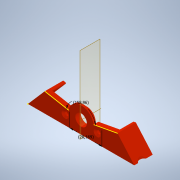
# Autodesk Inventor part: pizza_2
Saved by Autodesk Inventor 2022 (Build 260153000, 153)
## iProperties
Created: 2022-07-28
Part Number: pizza_2
Material: Типовые
Document SubType Name: Modeling
Designer: akapu
Density: 1 g/cm^3
Appearance: По умолчанию
Author: akapu
Autodesk Inventor part; units mm, degrees
ref_plane "YZ Plane" through (0, 0, 0) normal (1, 0, 0) x (0, 1, 0)
ref_plane "XZ Plane" through (0, 0, 0) normal (0, 1, 0) x (-1, 0, 0)
sketch "Эскиз1" plane through (0, 0, 0) normal (0, 0, 1) x (1, 0, 0)
  line L0 (0, 0) -> (35.556, 0)
  line L1 (35.556, 0) -> (57.84, 0)
  line L2 (57.84, 0) -> (93.396, 0)
  line L3 (0, 0) -> (67.4393, 0) construction
  line L4 (35.556, 0) -> (57.84, 0)
  line L5 (46.698, 0) -> (46.698, 11.142)
  line L6 (35.556, 0) -> (35.556, 11.142)
  line L7 (57.84, 0) -> (57.84, 11.142)
  circle A0 centre (46.698, 11.142) radius 11.142
  circle A1 centre (46.698, 11.142) radius 28
  line L8 (0, 0) -> (25.5349, 29.4757)
  line L9 (93.396, 0) -> (67.8611, 29.4757)
  line L10 (46.698, 11.142) -> (31.398, 11.142)
  line L11 (46.698, 11.142) -> (61.998, 11.142)
  circle A2 centre (31.398, 11.142) radius 1.6
  circle A3 centre (61.998, 11.142) radius 1.6
  line L12 (46.698, 11.142) -> (66.497, 30.941)
  line L13 (46.698, 11.142) -> (74.698, 11.142) construction
  line L14 (46.698, 11.142) -> (26.899, 30.941)
  line L15 (46.698, 11.142) -> (74.698, 11.142) construction
  line L16 (46.698, 11.142) -> (19.1687, 16.2546)
  line L17 (46.698, 11.142) -> (74.2273, 16.2546)
  line L18 (19.1687, 16.2546) -> (14.7865, 17.0684)
  line L19 (74.2273, 16.2546) -> (78.6095, 17.0684)
  point P0 (54.5766, 19.0206)
  point P1 (38.8194, 19.0206)
  point P2 (35.7433, 13.1764)
  point P3 (57.6527, 13.1764)
  dimension "d0" = 35.556
  dimension "d1" = 22.284
  dimension "d2" = 35.556
  dimension "d5" = 11.142
  dimension "d6" = 56
  dimension "d7" = 15.3
  dimension "d8" = 15.3
  dimension "d9" = 3.2
  dimension "d10" = 3.2
  dimension "d13" = 45
  dimension "d14" = 135
  constraints: 40 end point, 7 horizontal, 6 point on circle, 4 coincident, 4 point on line, 3 centre point, 3 vertical, 2 equal length, 2 tangent, 1 collinear, 1 midpoint, 3 other
  measures "d0" distance of L0.start L0.end
  measures "d1" distance of L0.end L1.end
  measures "d2" distance of L1.end L2.end
  measures "d5" distance of L5.start L5.end
  measures "d6" diameter of A1
  measures "d7" distance of L10.start L10.end
  measures "d8" distance of L10.start L11.end
  measures "d9" diameter of A2
  measures "d10" diameter of A3
  measures "d13" angle of L13 L12
  measures "d14" angle of L15 L14
extrude "Выдавливание1" add sketch "Эскиз1" along normal blind 2 contours L8 L18 A1 L0 | A1 L16 A0 L6 L0 | A1 L19 L9 L2 | L2 L7 A0 L17 A1 | A2 | A3
ref_plane "РабПлоскость2" through (-27.7885, -2.986, 3.8) normal (0, 0, 1) x (1, 0, 0)
sketch "Эскиз2" plane through (0, 0, 2) normal (0, 0, 1) x (1, 0, 0)
  circle A0 centre (46.698, 11.142) radius 11.1499
  line L0 (14.7865, 17.0684) -> (0, 0) projected
  line L1 (0, 0) -> (14.7865, 17.0684)
  line L2 (35.7433, 13.1764) -> (14.7865, 17.0684) projected
  line L3 (14.7865, 17.0684) -> (35.7433, 13.1764)
  line L4 (78.6095, 17.0684) -> (57.6527, 13.1764) projected
  line L5 (57.84, 0) -> (93.396, 0) projected
  line L6 (78.6095, 17.0684) -> (93.396, 0)
  line L7 (93.396, 0) -> (0, 0)
  line L8 (57.84, 11.142) -> (57.84, 0) projected
  arc A1 (57.84, 11.142) -> (57.6527, 13.1764) centre (46.698, 11.142) ccw projected
  line L9 (57.6527, 13.1764) -> (78.6095, 17.0684)
  line L10 (35.556, 0) -> (35.556, 11.142) projected
  line L11 (35.556, 0) -> (35.556, 8.243)
  line L12 (93.396, 0) -> (78.6095, 17.0684) projected
  line L13 (35.556, 0) -> (35.556, 8.257)
  line L14 (35.556, 8.257) -> (32.6, 8.257)
  point P0 (61.998, 11.142)
  point P1 (46.2772, 0)
  point P2 (47.1188, 0)
  point P3 (57.6605, 13.1779)
  point P4 (35.7355, 13.1779)
  dimension "d78" = 8.257
  dimension "d79" = 2.956
  constraints: 16 end point, 2 collinear, 2 point on line, 1 centre point, 1 horizontal, 1 perpendicular
  measures "d78" distance of L10.start L13.end
  measures "d79" distance of L13.end L14.end
extrude "Выдавливание2" add sketch "Эскиз2" along normal up to surface (1.8 mm away)
sketch "Эскиз5" plane through (0, 0, 0) normal (0, 0, -1) x (-1, 0, 0)
  line L0 (-35.7355, 13.1779) -> (-14.7865, 17.0684) projected
  line L1 (-14.7865, 17.0684) -> (-16.676, 15.4315)
  line L2 (-14.7865, 17.0684) -> (0, 0) projected
  line L3 (-16.676, 15.4315) -> (-3.3076, 0)
  line L4 (0, 0) -> (-46.2772, 0) projected
  line L5 (-16.676, 15.4315) -> (-17.6357, 16.5393)
  line L6 (-17.6357, 16.5393) -> (-14.7865, 17.0684)
  line L7 (-14.7865, 17.0684) -> (0, 0)
  line L8 (-3.3076, 0) -> (0, 0)
  line L9 (-93.396, 0) -> (-78.6095, 17.0684) projected
  line L10 (-78.6095, 17.0684) -> (-76.72, 15.4315)
  line L11 (-76.72, 15.4315) -> (-90.0884, 0)
  line L12 (-47.1188, 0) -> (-93.396, 0) projected
  line L13 (-93.396, 0) -> (-90.0884, 0)
  line L14 (-93.396, 0) -> (-78.6095, 17.0684)
  line L15 (-76.72, 15.4315) -> (-75.7603, 16.5393)
  line L16 (-78.6095, 17.0684) -> (-57.6605, 13.1779) projected
  line L17 (-78.6095, 17.0684) -> (-75.7603, 16.5393)
  dimension "d36" = 2.5
  dimension "d37" = 90
  dimension "d38" = 2.5
  dimension "d39" = 90
  constraints: 25 end point, 5 point on line, 3 collinear, 2 horizontal
  measures "d36" distance of L0.end L1.end
  measures "d37" angle of L2 L1
  measures "d38" distance of L9.end L10.end
  measures "d39" angle of L10 L9
extrude "Выдавливание5" add sketch "Эскиз5" along normal blind 12
sketch "Эскиз7" plane through (47.1188, 0, 2) normal (0, -1, 0) x (1, 0, 0)
  line L0 (-32.3324, 2) -> (-47.1188, 2) projected
  line L1 (-47.1188, 2) -> (-47.1188, -5)
  line L2 (-47.1188, -14) -> (-47.1188, 1.8) projected
  line L3 (-47.1188, -5) -> (-49.1188, -5)
  line L4 (0, 2) -> (46.2772, 2) projected
  line L5 (46.2772, 2) -> (46.2772, -5)
  line L6 (46.2772, 1.8) -> (46.2772, -14) projected
  line L7 (46.2772, -5) -> (48.2772, -5)
  circle A0 centre (-49.1188, -5) radius 3.5
  circle A1 centre (48.2772, -5) radius 4
  circle A2 centre (-49.1188, -5) radius 4
  point P0 (-47.1188, -2)
  dimension "d42" = 7
  dimension "d43" = 2
  dimension "d44" = 7
  dimension "d45" = 2
  dimension "d47" = 7
  dimension "d50" = 8
  dimension "d51" = 8
  constraints: 8 end point, 3 centre point, 3 coincident, 2 perpendicular, 2 point on line
  measures "d42" distance of L0.end L1.end
  measures "d43" distance of L1.end L3.end
  measures "d44" distance of L4.end L5.end
  measures "d45" distance of L5.end L7.end
  measures "d47" diameter of A0
  measures "d50" diameter of A1
  measures "d51" diameter of A2
extrude "Выдавливание6" cut sketch "Эскиз7" against normal blind 12
fillet "Сопряжение1" radius 0.5 2 edges at (17.6357, 16.5393, -6) (75.7603, 16.5393, -6)
sketch "Эскиз10" plane through (0, 0, 2) normal (0, 0, -1) x (-1, 0, 0)
  circle A0 centre (-46.698, 11.142) radius 1.5 projected
  circle A1 centre (-46.698, 11.142) radius 6
  circle A2 centre (-46.698, 11.142) radius 8
  point P0 (0, 0)
  dimension "d53" = 12
  dimension "d54" = 16
  constraints: 2 centre point, 2 coincident
  measures "d53" diameter of A1
  measures "d54" diameter of A2
extrude "Выдавливание7" add sketch "Эскиз10" along normal blind 3 contours A0 | A1 | A2
sketch "Эскиз11" plane through (46.698, 11.142, 2) normal (0, 0, -1) x (-1, 0, 0)
  circle A0 centre (0, 0) radius 1.5 projected
  circle A1 centre (0, 0) radius 5
  circle A2 centre (0, 0) radius 6
  point P0 (46.698, -11.142)
  constraints: 2 centre point, 2 coincident
extrude "Выдавливание8" cut sketch "Эскиз11" against normal blind 2 contours A0
ref_plane "РабПлоскость1" through (46.698, 11.142, 2) normal (1, 0, 0) x (0, 0, -1)
sketch "Эскиз15" plane through (0, 0, 0) normal (0, 0, -1) x (-1, 0, 0)
  line L0 (-57.84, 0) -> (-90.0884, 0) projected
  arc A0 (-76.3317, 15.8797) -> (-76.6184, 16.6986) centre (-76.7096, 16.207) ccw projected
  line L1 (-90.0884, 0) -> (-76.3317, 15.8797)
  circle A1 centre (-76.7096, 16.207) radius 0.5
  arc A2 (-57.6527, 13.1764) -> (-57.84, 11.142) centre (-46.698, 11.142) ccw projected
  line L2 (-76.6184, 16.6986) -> (-57.6527, 13.1764)
  line L3 (-90.0884, 0) -> (-76.3317, 15.8797) projected
  line L4 (-47.1188, 0) -> (-57.84, 0) projected
  line L5 (-90.0884, 0) -> (-57.84, 0)
  line L6 (-57.84, 11.142) -> (-57.84, 0) projected
  line L7 (-57.84, 0) -> (-57.84, 11.142)
  arc A3 (-35.556, 11.142) -> (-35.7433, 13.1764) centre (-46.698, 11.142) ccw projected
  line L8 (-35.556, 11.142) -> (-35.556, 0)
  line L9 (0, 0) -> (-46.2772, 0) projected
  line L10 (-3.3076, 0) -> (-17.0643, 15.8797) projected
  line L11 (-35.556, 0) -> (-3.3076, 0)
  line L12 (-3.3076, 0) -> (-17.0643, 15.8797)
  arc A4 (-35.7355, 13.1779) -> (-57.6605, 13.1779) centre (-46.698, 11.142) ccw projected
  line L13 (-35.7355, 13.1779) -> (-16.7776, 16.6986)
  arc A5 (-16.7776, 16.6986) -> (-17.0643, 15.8797) centre (-16.6864, 16.207) ccw projected
  circle A6 centre (-16.6864, 16.207) radius 0.5
  circle A7 centre (-46.698, 11.142) radius 11.142
  line L14 (-35.7355, 13.1779) -> (-35.7433, 13.1764)
  point P0 (-32.627, 8.243)
  constraints: 18 end point, 3 coincident, 2 collinear, 1 horizontal, 1 perpendicular, 1 point on line, 1 tangent, 1 vertical, 9 other
extrude "Выдавливание10" add sketch "Эскиз15" along normal blind 0.4 contours L0 L1 A0 L2 A2 L6 | A3 L14 L13 A5 L10 L9 L8
sketch "Эскиз16" plane through (0, 0, -12) normal (0, 0, -1) x (-1, 0, 0)
  line L0 (-35.7355, 13.1779) -> (-14.7865, 17.0684) projected
  line L1 (-14.7865, 17.0684) -> (0, 0)
  line L2 (-17.0643, 15.8797) -> (-3.3076, 0) projected
  line L3 (0, 0) -> (-3.3076, 0)
  line L4 (-3.3076, 0) -> (-17.0643, 15.8797)
  line L5 (-14.7865, 17.0684) -> (0, 0) projected
  arc A0 (-16.7776, 16.6986) -> (-17.0643, 15.8797) centre (-16.6864, 16.207) ccw projected
  line L6 (-14.7865, 17.0684) -> (-16.7776, 16.6986)
  line L7 (-90.0884, 0) -> (-76.3317, 15.8797) projected
  line L8 (-76.3317, 15.8797) -> (-90.0884, 0)
  line L9 (-93.396, 0) -> (-90.0884, 0) projected
  line L10 (-90.0884, 0) -> (-93.396, 0)
  line L11 (-78.6095, 17.0684) -> (-93.396, 0) projected
  line L12 (-93.396, 0) -> (-78.6095, 17.0684)
  arc A1 (-76.3317, 15.8797) -> (-76.6184, 16.6986) centre (-76.7096, 16.207) ccw projected
  line L13 (-78.6095, 17.0684) -> (-76.6184, 16.6986)
  circle A2 centre (-76.7096, 16.207) radius 0.5
  circle A3 centre (-16.6864, 16.207) radius 0.5
  constraints: 16 end point, 4 collinear, 2 coincident, 2 tangent, 1 horizontal, 6 other
extrude "Выдавливание11" add sketch "Эскиз16" along normal blind 0.4
sketch "Эскиз17" plane through (0, 0, -0.4) normal (0, 0, -1) x (-1, 0, 0)
  line L0 (-57.84, 0) -> (-57.84, 8.257)
  line L1 (-57.84, 11.142) -> (-57.84, 0) projected
  line L2 (-57.84, 8.257) -> (-35.556, 8.257)
  line L3 (-35.556, 0) -> (-35.556, 11.142) projected
  line L4 (-46.698, 8.257) -> (-60.7825, 8.257)
  line L5 (-46.698, 8.257) -> (-32.6135, 8.257)
  circle A0 centre (-60.7825, 8.257) radius 1.6
  circle A1 centre (-32.6135, 8.257) radius 1.6
  point P0 (0, 0)
  dimension "d83" = 8.257
  dimension "d84" = 14.0845
  dimension "d85" = 14.0845
  dimension "d86" = 3.2
  dimension "d87" = 3.2
  constraints: 8 end point, 4 point on line, 2 centre point, 2 coincident, 1 midpoint, 1 perpendicular
  measures "d83" distance of L0.start L0.end
  measures "d84" distance of L4.start L4.end
  measures "d85" distance of L4.start L5.end
  measures "d86" diameter of A0
  measures "d87" diameter of A1
extrude "Выдавливание12" cut sketch "Эскиз17" against normal blind 12
sketch "Эскиз18" plane through (0, 0, -0.4) normal (0, 0, -1) x (-1, 0, 0)
  circle A0 centre (-32.6135, 8.257) radius 1.6 projected
  circle A1 centre (-60.7825, 8.257) radius 1.6 projected
  point P0 (0, 0)
  dimension "d90" = 28.169
  measures "d90" distance of A0.centre A1.centre
chamfer "Фаска3" distance 1.5 angle 45 2 edges at (34.2135, 8.257, 3.8) (62.3825, 8.257, 3.8)
sketch "Эскиз20" plane through (0, 0, 3.8) normal (0, 0, 1) x (1, 0, 0)
  circle A0 centre (46.698, 11.142) radius 1.5 projected
  circle A1 centre (46.698, 11.142) radius 5.075
  point P0 (0, 0)
  dimension "d111" = 10.15
  constraints: 1 centre point, 1 coincident
  measures "d111" diameter of A1
extrude "Выдавливание14" cut sketch "Эскиз20" against normal blind 10 contours A0 | A1
sketch "Эскиз21" plane through (0, 0, 3.8) normal (0, 0, 1) x (1, 0, 0)
  line L0 (57.6605, 13.1779) -> (78.6095, 17.0684) projected
  line L1 (14.7865, 17.0684) -> (35.7355, 13.1779) projected
  point P0 (0, 0)
  dimension "d114" = 158.958
  measures "d114" angle of L0 L1
